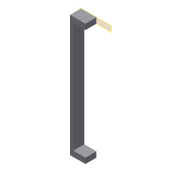
# Autodesk Inventor part: 06_OPENTRONS_Microscope_Extraslide
Saved by Autodesk Inventor 2019.4 (Build 234330000, 330)
## iProperties
Created: 2020-11-19
Part Number: 06_OPENTRONS_Microscope_Extraslide
Material: Generic
Document SubType Name: Modeling
Designer: diederichbenedict
Density: 1 g/cm^3
Appearance: Default
Author: diederichbenedict
Autodesk Inventor part; units mm, degrees
ref_plane "YZ Plane" through (0, 0, 0) normal (1, 0, 0) x (0, 1, 0)
ref_plane "XZ Plane" through (0, 0, 0) normal (0, 1, 0) x (-1, 0, 0)
ref_plane "XY Plane" through (0, 0, 0) normal (0, 0, 1) x (1, 0, 0)
ref_plane "Work Plane1" through (0, 0, 0) normal (0, 0, 1) x (1, 0, 0)
sketch "Sketch1" plane through (0, 0, 0) normal (0, 0, 1) x (1, 0, 0)
  line L0 (0, 0) -> (-19.6084, 0) projected
  line L1 (0, -10) -> (-19.6084, -10) projected
  line L2 (0, 0) -> (0, -10) projected
  line L3 (0, -210.5) -> (-19.6084, -210.5) projected
  line L4 (0, -220.5) -> (-19.6084, -220.5) projected
  line L5 (0, -220.5) -> (0, -210.5) projected
  line L6 (-52.6084, 0) -> (-46.6084, 0)
  line L7 (-46.6084, 0) -> (-46.6084, -220.5)
  line L8 (-46.6084, -220.5) -> (-52.6084, -220.5)
  line L9 (-52.6084, -220.5) -> (-52.6084, 0)
  line L10 (-35.1084, -220.5) -> (-35.1084, 29.5) construction
  line L11 (-29.1084, -220.5) -> (-29.1084, 29.5) construction
  line L12 (-46.6084, 0) -> (-24.6084, 0)
  line L13 (-24.6084, 0) -> (-24.6084, -10)
  line L14 (-24.6084, -10) -> (-46.6084, -10)
  line L15 (-46.6084, -10) -> (-46.6084, 0)
  line L16 (-46.6084, -220.5) -> (-24.6084, -220.5)
  line L17 (-24.6084, -220.5) -> (-24.6084, -210.5)
  line L18 (-24.6084, -210.5) -> (-46.6084, -210.5)
  line L19 (-46.6084, -210.5) -> (-46.6084, -220.5)
  line L20 (-19.6084, -10) -> (-19.6084, 0) projected
  line L21 (-19.6084, -220.5) -> (-19.6084, -210.5) projected
  dimension "d0" = 6
  dimension "d1" = 22
  dimension "d2" = 10
  dimension "d3" = 22
  dimension "d4" = 10
  constraints: 28 end point, 6 parallel, 3 horizontal, 3 perpendicular, 2 vertical, 1 point on line, 4 other
  measures "d0" distance of L7.end L8.end
  measures "d1" distance of L13.end L14.end
  measures "d2" distance of L12.end L13.end
  measures "d3" distance of L18.end L17.end
  measures "d4" distance of L17.end L16.end
extrude "Extrusion1" add sketch "Sketch1" along normal blind 20 contours L6 L7 L8 L9 | L12 L13 L14 L7 | L7 L18 L17 L16
sketch "Sketch2" plane through (-52.6084, 0, 0) normal (0, 1, 0) x (1, 0, 0)
  circle A0 centre (20.5, 120.1) radius 3 projected
  line L0 (0, 0) -> (28, 0) projected
  line L1 (0, 0) -> (0, -20) projected
  line L2 (28, -20) -> (0, -20) projected
  line L3 (28, 0) -> (28, -20) projected
  circle A1 centre (20.5, -10) radius 3.1
  point P0 (52.6084, 0)
  dimension "d7" = 6.2
  dimension "d8" = 10
  constraints: 1 centre point
  measures "d7" diameter of A1
  measures "d8" distance from line of A1.centre L0
extrude "Extrusion2" cut sketch "Sketch2" against normal through all contours A1
chamfer "Chamfer1" distance 10 angle 45 2 edges at (-46.6084, -10, 10) (-46.6084, -210.5, 10)
ref_plane "Work Plane2" through (0, 0, 10) normal (0, 0, 1) x (1, 0, 0)
body "Solid1"
